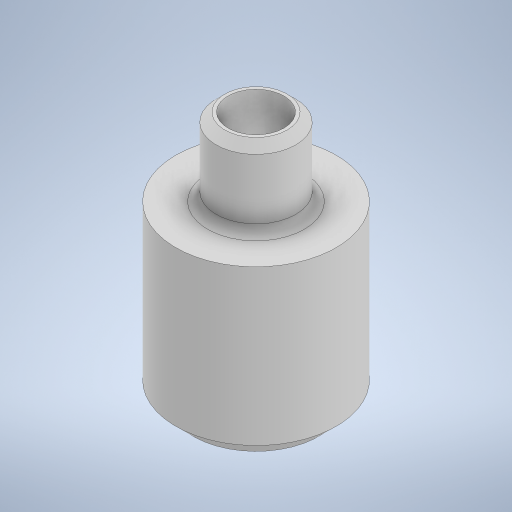
# Autodesk Inventor part: OutputFile
Saved by Autodesk Inventor 2024 (Build 280153000, 153)
## iProperties
Created: 2023-11-25
Part Number: OutputFile
Material: Genérico
Document SubType Name: Modeling
Designer: sergi
Density: 1 g/cm^3
Appearance: Valor por defecto
Mass: 4.87355 g
Surface Area: 26.8251 cm^2
Volume: 4.87355 cm^3
Author: sergi
Autodesk Inventor part; units mm, degrees
ref_plane "YZ Plane" through (0, 0, 0) normal (1, 0, 0) x (0, 1, 0)
ref_plane "XZ Plane" through (0, 0, 0) normal (0, 1, 0) x (-1, 0, 0)
ref_plane "XY Plane" through (0, 0, 0) normal (0, 0, 1) x (1, 0, 0)
sketch "Boceto1" plane through (0, 0, 0) normal (0, 1, 0) x (-1, 0, 0)
  circle A0 centre (0, 0) radius 9.325
  dimension "d0" = 18.65
  constraints: 1 centre point, 1 coincident
  measures "d0" diameter of A0
extrude "Extrusión1" add sketch "Boceto1" along normal blind 20
sketch "Boceto2" plane through (0, 20, 0) normal (0, 1, 0) x (1, 0, 0)
  circle A0 centre (0, 0) radius 4.625
  dimension "d3" = 9.25
  constraints: 1 centre point, 1 coincident
  measures "d3" diameter of A0
extrude "Extrusión2" add sketch "Boceto2" along normal blind 9
sketch "Boceto3" plane through (0, 29, 0) normal (0, 1, 0) x (1, 0, 0)
  circle A0 centre (0, 0) radius 4.625 projected
  constraints: 1 coincident
hole "Agujero1" at (0, 29, 0) direction (0, -1, 0) diameter 6.5 end through all
chamfer "Chaflán1" distance 2 angle 45 1 edges at (9.325, 0, 0)
chamfer "Chaflán2" distance 1 angle 45 1 edges at (-4.625, 29, 0)
fillet "Empalme1" radius 1 1 edges at (-4.625, 20, 0)
equation "\"d30\" = 0.125 * Sketch4_Pitch"
equation "\"Sketch4_Pitch\" = 1.5"
equation "\"d32\" = 60deg"
